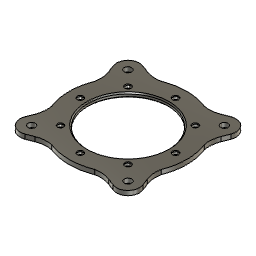
Assembly v1 (Autodesk Fusion 360 archive; units mm, degrees)
design "Motor_Base_Plate_Top v1"
Autodesk Fusion 360 part; units mm, degrees
sketch "Sketch1" plane through (0, 0, 0) normal (0, 0, 1) x (1, 0, 0)
  circle A0 centre (0, 0) radius 52.5
  line L0 (-52.5, 52.5) -> (52.5, 52.5)
  line L1 (52.5, 52.5) -> (52.5, -52.5)
  line L2 (52.5, -52.5) -> (-52.5, -52.5)
  line L3 (-52.5, -52.5) -> (-52.5, 52.5)
  line L4 (-52.5, 52.5) -> (52.5, -52.5) construction
  line L5 (52.5, 52.5) -> (-52.5, -52.5) construction
  circle A1 centre (0, 0) radius 42.5 construction
  circle A2 centre (0, 0) radius 35.75
  circle A3 centre (0, 42.5) radius 1.5
  circle A4 centre (-30.052, 30.052) radius 1.5
  circle A5 centre (-42.5, 0) radius 1.5
  circle A6 centre (-30.052, -30.052) radius 1.5
  circle A7 centre (0, -42.5) radius 1.5
  circle A8 centre (30.052, -30.052) radius 1.5
  circle A9 centre (42.5, 0) radius 1.5
  circle A10 centre (30.052, 30.052) radius 1.5
  dimension "d1" = 105
  dimension "d2" = 105
  dimension "d3" = 105
  dimension "d4" = 85
  dimension "d5" = 71.5
  dimension "d7" = 3
  dimension "d9" = 360
  constraint coincident A0.centre A1.centre
  constraint horizontal L0
  constraint perpendicular L0 L1
  constraint parallel L0 L2
  constraint parallel L1 L3
  constraint coincident L4 A0.centre
  constraint coincident L5 A0.centre
  constraint concentric A0 A1
  constraint coincident A1 A3.centre
  measures "d1" diameter of A0
  measures "d2" distance of L1.end L2.end
  measures "d3" distance of L0.end L1.end
  measures "d4" diameter of A1
  measures "d5" diameter of A2
  measures "d7" diameter of A3
extrude "Mounting_face_Extrude1" add sketch "Sketch1" along normal blind 4 contours A0
chamfer "Inner_hole_Chamfer" distance 1 angle 45 2 edges at (-33.3307, 12.9278, 4) (-33.3307, 12.9278, 0)
sketch "Sketch3" plane through (0, 0, 4) normal (0, 0, 1) x (-1, 0, 0)
  circle A0 centre (0, 0) radius 36.75
  circle A1 centre (0, 0) radius 52.5
  line L0 (0, 0) -> (37.1231, -37.1231) construction
  line L1 (0, 0) -> (52.5, 0) construction
  line L2 (54.8008, -19.4454) -> (19.4454, -54.8008) construction
  line L3 (37.1231, -37.1231) -> (49.3231, -37.1231) construction
  line L4 (37.1231, -37.1231) -> (28.4964, -45.7498)
  line L5 (28.4964, -45.7498) -> (45.7498, -28.4964)
  line L6 (45.7498, 28.4964) -> (28.4964, 45.7498)
  line L7 (19.4454, 54.8008) -> (54.8008, 19.4454) construction
  line L8 (-28.4964, 45.7498) -> (-45.7498, 28.4964)
  line L9 (-54.8008, 19.4454) -> (-19.4454, 54.8008) construction
  line L10 (-45.7498, -28.4964) -> (-28.4964, -45.7498)
  line L11 (-19.4454, -54.8008) -> (-54.8008, -19.4454) construction
  circle A2 centre (30.052, -30.052) radius 1.5
  circle A3 centre (42.5, 0) radius 1.5
  circle A4 centre (0, -42.5) radius 1.5
  circle A5 centre (30.052, 30.052) radius 1.5
  circle A6 centre (-42.5, 0) radius 1.5
  circle A7 centre (-30.052, -30.052) radius 1.5
  circle A8 centre (0, 42.5) radius 1.5
  circle A9 centre (-30.052, 30.052) radius 1.5
  circle A10 centre (42.5, 0) radius 2.75
  circle A11 centre (30.052, 30.052) radius 2.75
  circle A12 centre (0, 42.5) radius 2.75
  circle A13 centre (-30.052, 30.052) radius 2.75
  circle A14 centre (-42.5, 0) radius 2.75
  circle A15 centre (-30.052, -30.052) radius 2.75
  circle A16 centre (0, -42.5) radius 2.75
  circle A17 centre (30.052, -30.052) radius 2.75
  point P0 (28.4964, -45.7498)
  point P1 (45.7498, -28.4964)
  point P2 (45.7498, 28.4964)
  point P3 (28.4964, 45.7498)
  point P4 (-28.4964, 45.7498)
  point P5 (-45.7498, 28.4964)
  point P6 (-45.7498, -28.4964)
  point P7 (-28.4964, -45.7498)
  dimension "d24" = 45
  dimension "d26" = 25
  dimension "d31" = 12.2
  dimension "d71" = 360
  dimension "d115" = 5.5
  dimension "d117" = 360
  constraint horizontal L1
  constraint coincident A0.centre A1.centre
  constraint coincident A1 L0.end
  constraint symmetric L0 L2.start L2.end
  constraint horizontal L3
  constraint symmetric L3.start L0 L4.start
  constraint symmetric L0 P1 P0
  constraint coincident P0 L4.end
  constraint coincident P1 L5.end
  constraint concentric A3 A10
  measures "d24" angle of L0 L1
  measures "d26" distance of L0.end L2.start
  measures "d31" distance of L0.end P1
  measures "d115" diameter of A10
sketch "Sketch5" plane through (0, 0, 4) normal (0, 0, 1) x (1, 0, 0)
  line L0 (-45.7498, 28.4964) -> (-63.0032, 45.7498) construction
  line L1 (0, 0) -> (-37.1231, 37.1231)
  line L2 (-28.4964, 45.7498) -> (-45.7617, 62.9913) construction
  line L3 (-42.0139, 59.2438) -> (-59.2438, 42.0139) construction
  arc A0 (-42.0139, 59.2438) -> (-59.2438, 42.0139) centre (-50.6288, 50.6288) ccw construction
  arc A1 (-45.7617, 62.9913) -> (-63.0032, 45.7498) centre (-54.3825, 54.3706) ccw construction
  line L4 (-45.7617, 62.9913) -> (-42.0139, 59.2438) construction
  line L5 (-63.0032, 45.7498) -> (-59.2438, 42.0139) construction
  line L6 (-54.3765, 37.1231) -> (-50.0632, 32.8098) construction
  circle A2 centre (0, 0) radius 52.5 construction
  line L7 (-50.0632, 32.8098) -> (-48.8708, 19.1807) construction
  line L8 (-50.0632, 32.8098) -> (-41.1648, 32.8098) construction
  line L9 (-32.8098, 50.0632) -> (-19.1807, 48.8708) construction
  arc A3 (-48.8708, 19.1807) -> (-50.0632, 32.8098) centre (-73.2053, 23.9184) ccw
  arc A4 (-32.8098, 50.0632) -> (-19.1807, 48.8708) centre (-23.9184, 73.2053) ccw
  line L10 (-37.1231, 37.1231) -> (-42.9921, 42.9921) construction
  line L11 (-37.1231, 37.1231) -> (-18.8231, 37.1231) construction
  circle A5 centre (-42.9921, 42.9921) radius 3.3
  line L12 (-45.7498, 28.4964) -> (-44.7336, 27.4802) construction
  line L13 (-45.7498, 28.4964) -> (-44.3126, 28.4964) construction
  line L14 (-28.4964, 45.7498) -> (-27.4802, 44.7336) construction
  arc A6 (-27.4802, 44.7336) -> (-48.8708, 19.1807) centre (0, 0) ccw construction
  arc A7 (-19.1807, 48.8708) -> (-48.8708, 19.1807) centre (0, 0) ccw
  line L15 (-52.5, 0) -> (-71.6, 0) construction
  line L16 (-50.0632, 32.8098) -> (-52.5813, 39.2323)
  line L17 (-32.8098, 50.0632) -> (-39.2323, 52.5813)
  arc A8 (-39.2323, 52.5813) -> (-52.5813, 39.2323) centre (-42.9921, 42.9921) ccw
  line L18 (-50.0632, -32.8098) -> (-52.5813, -39.2323)
  arc A9 (-50.0632, -32.8098) -> (-48.8708, -19.1807) centre (-73.2053, -23.9184) ccw
  arc A10 (-44.7336, -27.4802) -> (-19.1807, -48.8708) centre (0, 0) ccw construction
  arc A11 (-48.8708, -19.1807) -> (-19.1807, -48.8708) centre (0, 0) ccw
  arc A12 (-19.1807, -48.8708) -> (-32.8098, -50.0632) centre (-23.9184, -73.2053) ccw
  line L19 (-32.8098, -50.0632) -> (-39.2323, -52.5813)
  arc A13 (-52.5813, -39.2323) -> (-39.2323, -52.5813) centre (-42.9921, -42.9921) ccw
  circle A14 centre (-42.9921, -42.9921) radius 3.3
  line L20 (-37.1231, -37.1231) -> (-42.9921, -42.9921) construction
  line L21 (32.8098, -50.0632) -> (39.2323, -52.5813)
  arc A15 (32.8098, -50.0632) -> (19.1807, -48.8708) centre (23.9184, -73.2053) ccw
  arc A16 (27.4802, -44.7336) -> (48.8708, -19.1807) centre (0, 0) ccw construction
  arc A17 (19.1807, -48.8708) -> (48.8708, -19.1807) centre (0, 0) ccw
  arc A18 (48.8708, -19.1807) -> (50.0632, -32.8098) centre (73.2053, -23.9184) ccw
  line L22 (50.0632, -32.8098) -> (52.5813, -39.2323)
  arc A19 (39.2323, -52.5813) -> (52.5813, -39.2323) centre (42.9921, -42.9921) ccw
  circle A20 centre (42.9921, -42.9921) radius 3.3
  line L23 (37.1231, -37.1231) -> (42.9921, -42.9921) construction
  line L24 (50.0632, 32.8098) -> (52.5813, 39.2323)
  arc A21 (50.0632, 32.8098) -> (48.8708, 19.1807) centre (73.2053, 23.9184) ccw
  arc A22 (44.7336, 27.4802) -> (19.1807, 48.8708) centre (0, 0) ccw construction
  arc A23 (48.8708, 19.1807) -> (19.1807, 48.8708) centre (0, 0) ccw
  arc A24 (19.1807, 48.8708) -> (32.8098, 50.0632) centre (23.9184, 73.2053) ccw
  line L25 (32.8098, 50.0632) -> (39.2323, 52.5813)
  arc A25 (52.5813, 39.2323) -> (39.2323, 52.5813) centre (42.9921, 42.9921) ccw
  circle A26 centre (42.9921, 42.9921) radius 3.3
  line L26 (37.1231, 37.1231) -> (42.9921, 42.9921) construction
  line L27 (71.1, 0) -> (50.5, 0) construction
  point P0 (-45.7498, 28.4964)
  point P1 (-59.2438, 59.2438)
  point P2 (-50.0632, 32.8098)
  point P3 (-54.3765, 37.1231)
  point P4 (-85.5492, 19.4221)
  point P5 (-32.8098, 50.0632)
  point P6 (-37.1231, 54.3765)
  point P7 (-32.8098, 50.0632)
  point P8 (-50.6288, 50.6288)
  point P9 (-52.5, 0)
  point P10 (-50.2753, 50.2753)
  point P11 (-37.1231, 37.1231)
  point P12 (-50.2753, -50.2753)
  point P13 (-48.8708, -19.1807)
  point P14 (-50.0632, -32.8098)
  point P15 (-32.8098, -50.0632)
  point P16 (50.2753, -50.2753)
  point P17 (19.1807, -48.8708)
  point P18 (32.8098, -50.0632)
  point P19 (50.0632, -32.8098)
  point P20 (50.2753, 50.2753)
  point P21 (48.8708, 19.1807)
  point P22 (50.0632, 32.8098)
  point P23 (32.8098, 50.0632)
  dimension "d36" = 6.1
  dimension "d37" = 85
  dimension "d38" = 135
  dimension "d39" = 8.3
  dimension "d40" = 6.6
  dimension "d41" = 45
  dimension "d65" = 19.1
  dimension "d94" = 18.6
  dimension "d96" = 360
  dimension "d97" = 20.6
  constraint coincident P0 L0.start
  constraint symmetric P0 L1 L2.start
  constraint symmetric L3.end L1 L3.start
  constraint midpoint L3 A0.centre
  constraint midpoint A0 P1
  constraint midpoint L0 P3
  constraint coincident P2 L6.end
  constraint horizontal L8
  constraint coincident A2 L7.end
  constraint coincident P3 L6.start
  constraint symmetric L1 P2 P7
  constraint symmetric L1 L7.end L9.end
  constraint symmetric L1 P3 P6
  constraint coincident P2 A3
  constraint symmetric L1 A3 A4
  constraint horizontal L11
  constraint coincident P11 L1.end
  constraint coincident P7 P5
  constraint coincident L10.end A5.centre
  constraint horizontal L13
  constraint coincident A2 L12.end
  constraint symmetric L10 P0 L2.start
  constraint symmetric L10 L12.end L14.end
  constraint coincident P11 A6
  constraint coincident P11 A7
  constraint coincident A0.centre P8
  constraint coincident P9 L15.start
  constraint concentric A5 A8
  constraint tangent L16 A8
  constraint symmetric L10 P2 P7
  constraint symmetric L10 L16.end L17.end
  constraint midpoint A8 P10
  constraint horizontal L27
  measures "d36" distance of P3 P2
  measures "d37" angle of L7 L8
  measures "d38" angle of L10 L11
  measures "d39" distance of P11 L10.end
  measures "d40" diameter of A5
  measures "d41" angle of L12 L13
  measures "d65" distance of P9 L15.end
  measures "d94" distance of P10 P11
  measures "d97" distance of L27.start L27.end
extrude "Extrude6" add sketch "Sketch5" against normal blind 4
chamfer "Chamfer4" distance 0.5 angle 45 8 edges at (28.6535, 30.5945, 4) (-1.3985, 43.0424, 4) (41.1015, 0.5424, 4) (28.6535, -29.5096, 4) (-1.3985, -41.9576, 4) (-31.4505, -29.5096, 4) (-43.8985, 0.5424, 4) (-31.4505, 30.5945, 4)
extrude "Extrude9" cut sketch "Sketch3" against normal blind 1 contours A10 | A11 | A12 | A13 | A14 | A15 | A16 | A17
chamfer "Chamfer5" distance 1.25 angle 45 8 edges at (-1.3985, 41.9576, 3) (-31.4505, 29.5096, 3) (-31.4505, -30.5945, 3) (-43.8985, -0.5424, 3) (-1.3985, -43.0424, 3) (28.6535, -30.5945, 3) (41.1015, -0.5424, 3) (28.6535, 29.5096, 3)
equation "d31 = ( 36.6 / 3 ) * 1 mm"
equation "d36 = 12.200 mm / 2"
equation "d39 = 5 mm + 3.3 mm"
equation "d97 = 10.300 mm * 2"

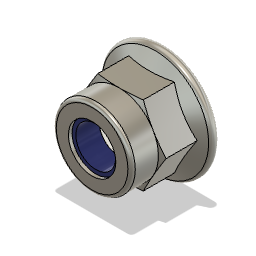
design "Prevailing Torque Type Hexagon Nut ČSN EN 1663 - M6 Steel 6 Plain"
description: Prevailing Torque Type Hexagon Nut ČSN EN 1663 - M6
Autodesk Fusion 360 part; units mm, degrees
sketch "Sketch1" plane through (0, 0, 0) normal (0, 1, 0) x (1, 0, 0)
  line L0 (0, 0) -> (0, -9.1)
  line L1 (-3, 0) -> (-5.775, 0)
  line L2 (-5.775, 0) -> (-5.775, -5.4923)
  line L3 (-5.775, -5.4923) -> (-5, -5.7)
  line L4 (-5, -5.7) -> (-5, -8.638)
  line L5 (-4.538, -9.1) -> (-3, -9.1)
  line L6 (-3, -9.1) -> (-3, -8.638)
  line L7 (-3, -8.638) -> (-4.538, -8.638)
  line L8 (-4.538, -8.638) -> (-4.538, -5.7)
  line L9 (-4.538, -5.7) -> (-3, -5.7)
  line L10 (-3, 0) -> (-3, -5.7)
  arc A0 (-5, -8.638) -> (-4.538, -9.1) centre (-4.538, -8.638) ccw
  point P0 (-5, -9.1)
  dimension "d127" = 11.55
  dimension "d140" = 10
  dimension "d148" = 5.7
  dimension "d150" = 6
  dimension "d151" = 9.1
  dimension "d152" = 6
  dimension "d153" = 0.462
  dimension "d154" = 0.462
  dimension "d182" = 15
  dimension "d191" = 9.1
  constraint vertical L0
  constraint vertical L2
  constraint coincident L0.start origin
  constraint coincident L0.start L1
  constraint horizontal L1
  constraint perpendicular L4 L5
  constraint perpendicular L5 L6
  constraint perpendicular L6 L7
  constraint vertical L10
  constraint horizontal L9
  constraint horizontal L3.end L8.end
  constraint vertical L6
  constraint coincident P0 L4
  constraint coincident P0 L5
  constraint tangent L4 A0
  constraint tangent L5 A0
  constraint coincident L7.end L8.start
  measures "d148" distance of L1 L3.end
  measures "d151" distance of L1 P0
  measures "d153" distance of L5.end L6.end
  measures "d154" distance of L4 L8
  measures "d182" angle of L3 L9
  measures "d191" distance of L0.start L0.end
revolve "Revolve4" add sketch "Sketch1" angle 360 about axis through (0, 0, 0) along (0, 0, 1) makes body 1
sketch "Sketch15" plane through (0, 0, 9.1) normal (0, 0, 1) x (1, 0, 0)
  circle A0 centre (0, 0) radius 3
  line L0 (0, 0) -> (2.8868, 5)
  line L1 (0, 0) -> (-2.8868, 5)
  line L2 (-2.8868, 5) -> (2.8868, 5)
  line L3 (0, 0) -> (0, 10) construction
  line L4 (-2.8868, 5) -> (2.8868, 5)
  line L5 (2.8868, 5) -> (2.8868, 5.8328)
  line L6 (2.8868, 5.8327) -> (-2.8868, 5.8327)
  line L7 (-2.8868, 5.8327) -> (-2.8868, 5)
  circle A1 centre (0, 0) radius 4.538
  dimension "d158" = 60
  dimension "d159" = 60
  dimension "d160" = 5
  dimension "d161" = 5.8327
  constraint coincident A0.centre L0.start
  constraint vertical L3
  constraint midpoint L2 L3
  constraint horizontal L4
  constraint vertical L5
  constraint horizontal L6
  constraint vertical L7
  constraint coincident L0.end L2.end
  measures "d158" angle of L0 L1
  measures "d159" angle of L0 L2
  measures "d160" distance of A0.centre L2
  measures "d161" distance of A0.centre L6
extrude "Extrude12" cut sketch "Sketch15" against normal through all contours L2 L4 L5 L6 L7 bodies 1
pattern_circular "C-Pattern3" count 6 over 360 about axis through (0, 0, 1.75) along (0, 0, 1) of "Extrude12"
thread "Thread4" "ISO Metric profile 6.0 M6x1 6H" major diameter 6.147 minor diameter 5.035 pitch 1 angle 60 resizes the face on face at (-2.9963, 0.1495, 1.9) on bodies 1
sketch "Sketch16" plane through (0, 0, 0) normal (0, 1, 0) x (1, 0, 0)
  line L0 (-4.538, -8.638) -> (-4.538, -5.7)
  line L1 (-4.538, -5.7) -> (-3, -5.7)
  line L2 (-3, -8.638) -> (-4.538, -8.638)
  line L3 (2.5175, -5.7) -> (-2.5175, -5.7)
  line L4 (-4.538, -8.638) -> (-2.5175, -8.638)
  line L5 (-2.5175, -8.638) -> (-2.5175, -5.7)
  line L6 (-2.5175, -5.7) -> (-4.538, -5.7)
  line L7 (-4.538, -5.7) -> (-4.538, -8.638)
  constraint horizontal L4
  constraint vertical L5
  constraint horizontal L6
  constraint vertical L7
  constraint coincident L3.end L5.end
  constraint coincident L0.start L2.end
revolve "Revolve5" add sketch "Sketch16" angle 360 about axis through (0, 0, 0) along (0, 0, 1) separate body makes body 2
sketch "Sketch17" plane through (0, 0, 0) normal (0, 1, 0) x (1, 0, 0)
  arc A0 (-6.523, 0) -> (-6.7668, -1.1) centre (-6.523, -0.577) ccw
  line L0 (-6.523, -0.577) -> (-7.1, -0.577) construction
  line L1 (-6.7668, -1.1) -> (-4.5, -2.157)
  line L2 (-4.5, -2.157) -> (-4.5, 0)
  line L3 (0, 0) -> (0, -9.1)
  line L4 (-6.523, 0) -> (0, 0)
  dimension "d181" = 1.1
  dimension "d192" = 9
  dimension "d193" = 14.2
  dimension "d194" = 25
  constraint coincident A0.centre L0.start
  constraint tangent A0 L1
  constraint coincident A0 L1.start
  constraint horizontal L0
  constraint coincident A0.end L1.start
  constraint coincident A0 L0.end
  constraint tangent A0 L4
  constraint perpendicular L3 L4
  constraint coincident L2.end L4
  constraint perpendicular L2 L4
  constraint coincident L3.start L4.end
  measures "d181" vertical distance of A0.start A0.end
  measures "d194" angle of L1 L4
revolve "Revolve6" add sketch "Sketch17" angle 360 about axis through (0, 0, 1.75) along (0, 0, 1) bodies 1
equation "adsk_nheig = 9.10 mm"
equation "adsk_wacor = 11.55 mm"
equation "adsk_nomdia = 6.00 mm"
equation "adsk_waflat = 10.00 mm"
equation "d127 = adsk_wacor"
equation "adsk_bheig = 5.70 mm"
equation "d140 = adsk_waflat"
equation "adsk_chamang2 = 15.00 deg"
equation "d148 = adsk_bheig"
equation "d150 = adsk_nomdia"
equation "d151 = adsk_nheig"
equation "d152 = adsk_nomdia"
equation "d153 = adsk_wacor * 0.04"
equation "d154 = d153"
equation "d160 = adsk_waflat / 2"
equation "d161 = adsk_wacor / 2 * 1.01"
equation "adsk_maxdia = 14.20 mm"
equation "adsk_flngheig = 1.10 mm"
equation "adsk_flngang = 25.00 deg"
equation "d181 = adsk_flngheig"
equation "d182 = adsk_chamang2"
equation "d189 = adsk_nheig"
equation "d191 = adsk_nheig"
equation "d192 = adsk_waflat * 0.9"
equation "d193 = adsk_maxdia"
equation "d194 = adsk_flngang"

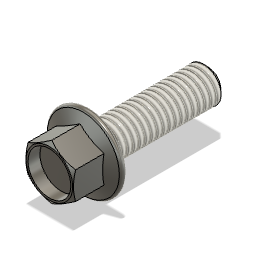
design "Indented Hex Flange Head Machine Screw ANSI B18.6.7M - M6x1 x 20 Steel Grade 2 Plain"
description: Indented Hex Flange Head Machine Screw ANSI B18.6.7M - M6x1 x 20
Autodesk Fusion 360 part; units mm, degrees
sketch "Sketch1" plane through (0, 0, 0) normal (0, 1, 0) x (1, 0, 0)
  line L0 (-3, 0) -> (-3, 20)
  line L1 (-3, 20) -> (0, 20)
  line L2 (0, 20) -> (0, -4.7)
  line L3 (-3, 0) -> (-4.62, 0)
  line L4 (-4.62, 0) -> (-4.62, -6.2959)
  line L5 (-3.92, -6.7) -> (-3.6, -6.7)
  line L6 (-3.92, -6.7) -> (-4.62, -6.2959)
  line L7 (-3.6, -6.7) -> (-3.6, -4.7)
  line L8 (-3.6, -4.7) -> (0, -4.7)
  dimension "d9" = 6
  dimension "d68" = 20
  dimension "d111" = 6.7
  dimension "d113" = 30
  dimension "d114" = 9.24
  dimension "d115" = 7.84
  dimension "d158" = 7.2
  dimension "d159" = 2
  constraint perpendicular L0 L1
  constraint perpendicular L0 L3
  constraint coincident origin L3
  constraint vertical L0
  constraint vertical L2
  constraint parallel L2 L4
  constraint coincident L2 L8.end
  constraint perpendicular L2 L5
  constraint coincident L3.end L4.start
  constraint perpendicular L5 L7
  constraint perpendicular L2 L8
  constraint coincident L2.end L8.end
  constraint coincident origin L2
  measures "d68" distance of origin L1.end
  measures "d111" distance of L3 L5
  measures "d113" angle of L5 L6
  measures "d159" distance of L5.end L7.end
revolve "Revolve1" add sketch "Sketch1" angle 360 about axis through (0, 0, -20) along (0, 0, 1)
sketch "Sketch8" plane through (0, 0, 0) normal (0, 0, 1) x (1, 0, 0)
  line L0 (0, 0) -> (-4, 0) construction
  line L1 (-4, -2.3118) -> (-4, 2.3118)
  circle A0 centre (0, 0) radius 4.62
  dimension "d110" = 4
  constraint horizontal L0
  constraint perpendicular L0 L1
  constraint coincident L0.end L1
  constraint coincident L0.start A0.centre
  constraint coincident L1.end A0
  constraint coincident L1.start A0
  measures "d110" distance of L0.start L1
extrude "Extrude5" cut sketch "Sketch8" along normal blind 6.7 contours L1 A0 picked at (-4.1, -0.5631)
pattern_circular "C-Pattern2" count 6 over 360 about axis through (0, 0, 1.75) along (0, 0, 1) of "Extrude5"
sketch "Sketch12" plane through (0, 0, 0) normal (0, 1, 0) x (1, 0, 0)
  line L0 (3.8, 0) -> (5.8845, 0)
  line L1 (6.0608, -1) -> (3.8, -1.8229)
  line L2 (3.8, -1.8229) -> (3.8, 0)
  arc A0 (6.0608, -1) -> (5.8845, 0) centre (5.8845, -0.5155) ccw
  line L3 (0, -1.75) -> (0, -22.5)
  line L4 (4.62, 0) -> (4.62, -1.5244) construction
  line L5 (0, 0) -> (4, 0)
  line L6 (6.4, 0) -> (6.4, -1.8229) construction
  line L7 (3.8, -1.8229) -> (6.4, -1.8229) construction
  dimension "d122" = 7.6
  dimension "d126" = 9.24
  dimension "d138" = 1
  dimension "d142" = 6.4
  dimension "d163" = 20
  constraint horizontal L0
  constraint perpendicular L0 L2
  constraint tangent L0 A0
  constraint tangent L1 A0
  constraint horizontal L5.start L0.start
  constraint coincident L1 L4.end
  constraint perpendicular L0 L4
  constraint coincident L0 L4.start
  constraint vertical L6
  constraint tangent A0 L6
  constraint coincident L0 L6.start
  constraint perpendicular L6 L7
  constraint coincident L6.end L7.end
  measures "d138" vertical distance of L0.end L1.start
  measures "d142" distance of L5.start L6
  measures "d163" angle of L0 L1
revolve "Revolve3" add sketch "Sketch12" angle 360 about axis through (0, 0, 1.75) along (0, 0, 1)
thread "Thread2" "ISO Metric profile 6.0 M6x1 6g" major diameter 5.884 minor diameter 4.7435 pitch 1 angle 60 resizes the face on face at (-2.9851, 0.2987, -6.6667) from (0, 0, -2.3) to (0, 0, -20)
fillet "Fillet4" radius 0.2 1 edges at (2.7429, -1.0639, 0)
sketch "Sketch5" plane through (0, 0, 0) normal (0, 1, 0) x (1, 0, 0)
  line L0 (-3.06, 19.125) -> (-2.125, 20)
  line L1 (0, -1.75) -> (0, -22.5)
  line L2 (0, 20) -> (0, -4.7)
  line L3 (0, 20) -> (-3.06, 20)
  line L4 (-3.06, 20) -> (-3.06, 19.125)
  dimension "d153" = 2.125
  dimension "d156" = 3.06
  dimension "d157" = 0.875
  constraint coincident L2.start L3.start
  constraint perpendicular L2 L3
  constraint coincident L0.end L3
  constraint perpendicular L3 L4
  measures "d153" distance of L0.end L1
  measures "d156" horizontal distance of origin L3.end
  measures "d157" distance of L0.start L3.end
revolve "Revolve2" cut sketch "Sketch5" angle 360 about axis through (0, 0, -20) along (0, 0, 1)
equation "d9 = adsk_nomdia"
equation "adsk_nomlen = 20.00 mm"
equation "adsk_headh = 6.70 mm"
equation "adsk_nomdia = 6.00 mm"
equation "d68 = adsk_nomlen"
equation "d89 = adsk_headh"
equation "adsk_waflat = 8.00 mm"
equation "d110 = adsk_waflat / 2"
equation "d111 = adsk_headh"
equation "d113 = adsk_chamang2"
equation "d114 = adsk_wacor"
equation "d115 = adsk_topdia"
equation "d122 = adsk_waflat * 0.95"
equation "d126 = adsk_waflat * 1.155"
equation "adsk_headdia = 12.80 mm"
equation "adsk_flngheig = 1.00 mm"
equation "adsk_thrlen = 17.70 mm"
equation "d133 = adsk_nomdia / 30"
equation "d138 = adsk_flngheig"
equation "d142 = adsk_headdia / 2"
equation "d144 = adsk_thrlen"
equation "adsk_endpointdia = 4.25 mm"
equation "d153 = adsk_endpointdia / 2"
equation "adsk_startlen = 0.875 mm"
equation "d156 = adsk_nomdia * 0.51"
equation "d157 = adsk_startlen"
equation "d158 = adsk_indentdia"
equation "d159 = adsk_indentdepth"
equation "adsk_wacor = 9.24 mm"
equation "adsk_topdia = adsk_waflat * 0.98"
equation "adsk_chamang2 = 30.00 deg"
equation "d163 = adsk_flngang"
equation "adsk_flngang = 20.00 deg"
equation "adsk_indentdia = 7.20 mm"
equation "adsk_indentdepth = 2.00 mm"
